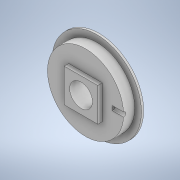
# Autodesk Inventor part: Motorstange_version2a
Saved by Autodesk Inventor 2021 (Build 250183000, 183)
## iProperties
Created: 2022-06-26
Part Number: Motorstange_version2a
Material: Generisch
Document SubType Name: Modeling
Designer: adria
Mass: 5.58467 g
Surface Area: 33.9161 cm^2
Volume: 5.58467 cm^3
Density: 1 g/cm^3
Appearance: Vorgabe
Author: adria
Autodesk Inventor part; units mm, degrees
ref_plane "XZ Plane" through (0, 0, 0) normal (0, 1, 0) x (-1, 0, 0)
ref_plane "XY Plane" through (0, 0, 0) normal (0, 0, 1) x (1, 0, 0)
sketch "Skizze1" plane through (0, 0, 0) normal (0, 0, 1) x (1, 0, 0)
  circle A0 centre (0, 0) radius 20
  dimension "d0" = 40
  constraints: 1 centre point, 1 coincident
  measures "d0" diameter of A0
extrude "Extrusion1" add sketch "Skizze1" along normal blind 1
sketch "Skizze2" plane through (0, 0, 1) normal (0, 0, 1) x (1, 0, 0)
  circle A0 centre (0, 0) radius 20 projected
  circle A1 centre (0, 0) radius 17
  dimension "d3" = 34
  constraints: 1 centre point, 1 coincident
  measures "d3" diameter of A1
extrude "Extrusion2" add sketch "Skizze2" along normal blind 10 contours A1
sketch "Skizze3" plane through (0, 0, 11) normal (0, 0, 1) x (1, 0, 0)
  circle A0 centre (0, 0) radius 17 projected
  circle A1 centre (0, 0) radius 20
  dimension "d6" = 40
  constraints: 1 centre point, 1 coincident
  measures "d6" diameter of A1
extrude "Extrusion3" add sketch "Skizze3" along normal blind 1 contours A0 | A1
sketch "Skizze6" plane through (0, 0, 12) normal (0, 0, 1) x (1, 0, 0)
  circle A0 centre (0, 0) radius 20 projected
  circle A1 centre (0, 0) radius 5.1
  dimension "d16" = 10.2
  constraints: 1 centre point, 1 coincident
  measures "d16" diameter of A1
extrude "Extrusion6" cut sketch "Skizze6" against normal through all contours A1
sketch "Skizze7" plane through (0, 0, 0) normal (0, 1, 0) x (-1, 0, 0)
  line L0 (17, 1) -> (17, 11) projected
  line L1 (-17, 1) -> (-17, 11) projected
  line L2 (20, 0) -> (-20, 0) projected
  line L3 (20, 0) -> (20, 1) projected
  line L4 (20, 1) -> (-20, 1) projected
  line L5 (-17, 1) -> (-17, 11) projected
  line L6 (20, 0) -> (-20, 0)
  line L7 (-20, 0) -> (-20, 6)
  line L8 (-20, 6) -> (20, 6)
  line L9 (20, 6) -> (20, 0)
  line L10 (20, 12) -> (-20, 12) projected
  point P0 (0, 0)
  dimension "d19" = 6
  dimension "d20" = 12
  constraints: 8 end point, 2 parallel, 1 horizontal, 1 perpendicular
  measures "d19" distance between parallel lines of L8 L10
  measures "d20" distance between parallel lines of L10 L2
extrude "Extrusion7" cut sketch "Skizze7" along normal through all both and the other way through all keep common part
ref_plane "Arbeitsebene2" through (17, 0, 0) normal (1, 0, 0) x (0, 1, 0)
sketch "Skizze9" plane through (17, 0, 0) normal (1, 0, 0) x (0, 1, 0)
  line L0 (17, 6) -> (-17, 6) projected
  circle A0 centre (0, 6) radius 1
  point P0 (0, 0)
  point P1 (-1, 6)
  point P2 (1, 6)
  dimension "d24" = 2
  constraints: 1 centre point, 1 midpoint
  measures "d24" diameter of A0
extrude "Extrusion8" cut sketch "Skizze9" against normal blind 5 contours A0 L0 picked at (0.0402, 5.6691)
sketch "Skizze10" plane through (12, 1, 6) normal (0, 0, 1) x (1, 0, 0)
  circle A0 centre (-12, -1) radius 5.1 projected
  line L0 (-19.5, 6.5) -> (-4.5, 6.5)
  line L1 (-4.5, 6.5) -> (-4.5, -8.5)
  line L2 (-4.5, -8.5) -> (-19.5, -8.5)
  line L3 (-19.5, -8.5) -> (-19.5, 6.5)
  line L4 (-19.5, 6.5) -> (-4.5, -8.5) construction
  line L5 (-4.5, 6.5) -> (-19.5, -8.5) construction
  dimension "d27" = 15
  dimension "d28" = 15
  constraints: 12 end point, 2 midpoint, 2 parallel, 1 horizontal, 1 perpendicular
  measures "d27" distance of L0.start L0.end
  measures "d28" distance of L0.end L1.end
extrude "Extrusion9" add sketch "Skizze10" along normal blind 2
equation "\"d19\" = 0.5 * d20"
equation "\"d28\" = d27"
